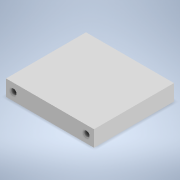
# Autodesk Inventor part: Stepper Standoff
Saved by Autodesk Inventor 2020 (Build 240168000, 168)
## iProperties
Created: 2020-03-20
Part Number: Stepper Standoff
Material: Generic
Document SubType Name: Modeling
Designer: DasNick
Density: 1 g/cm^3
Appearance: Default
Author: DasNick
Autodesk Inventor part; units mm, degrees
ref_plane "YZ Plane" through (0, 0, 0) normal (1, 0, 0) x (0, 1, 0)
ref_plane "XZ Plane" through (0, 0, 0) normal (0, 1, 0) x (-1, 0, 0)
ref_plane "XY Plane" through (0, 0, 0) normal (0, 0, 1) x (1, 0, 0)
sketch "Sketch1" plane through (0, 0, 0) normal (0, 0, 1) x (1, 0, 0)
  circle A0 centre (29.0032, 44.45) radius 2.3813 projected
  circle A1 centre (-29.0032, 44.45) radius 2.3813 projected
  circle A2 centre (29.0032, -44.45) radius 2.3813 projected
  circle A3 centre (29.0032, 44.45) radius 2.3813 projected
  circle A4 centre (-29.0032, -44.45) radius 2.3813 projected
  circle A5 centre (-29.0032, 44.45) radius 2.3813 projected
  circle A6 centre (0, 0) radius 14.2875 projected
  circle A7 centre (30.1625, -19.05) radius 2.3813 projected
  circle A8 centre (30.1625, 0) radius 2.3813 projected
  circle A9 centre (30.1625, 19.05) radius 2.3813 projected
  line L0 (-34.925, -65.8813) -> (34.925, -65.8812) projected
  line L1 (34.925, 65.8813) -> (-34.925, 65.8812) projected
  line L2 (-34.925, 65.8812) -> (-34.925, -65.8813) projected
  circle A10 centre (30.1625, -59.5312) radius 2.3813 projected
  circle A11 centre (30.1625, 59.5313) radius 2.3813 projected
  circle A12 centre (-30.1625, 59.5312) radius 2.3813 projected
  circle A13 centre (-30.1625, -59.5313) radius 2.3813 projected
  line L3 (34.925, 50.8) -> (-34.925, 50.8)
  line L4 (-34.925, 50.8) -> (-34.925, 38.1)
  line L5 (-34.925, 38.1) -> (34.925, 38.1)
  line L6 (34.925, 38.1) -> (34.925, 50.8)
  point P0 (0, 0)
  point P1 (-34.925, 50.8)
  dimension "d0" = 12.7
  dimension "d3" = 6.35
  constraints: 8 end point, 2 parallel, 1 horizontal, 1 perpendicular, 1 point on line
  measures "d0" distance of L5.end L3.start
  measures "d3" distance from line of L3 A0.centre
extrude "Extrusion1" add sketch "Sketch1" along normal blind 63.5 contours L3 L6 L5 L2
body "Solid1"
